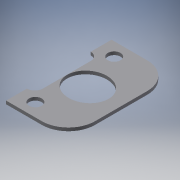
# Autodesk Inventor part: mocowanie_podwozia_dol
Saved by Autodesk Inventor 2017 (Build 210142000, 142)
## iProperties
Created: 2017-05-12
Part Number: mocowanie_podwozia_dol
Material: Ogólny
Document SubType Name: Modeling
Designer: Kuba01
Density: 1 g/cm^3
Appearance: Domyślna
Author: Kuba01
Autodesk Inventor part; units mm, degrees
ref_plane "YZ Plane" through (0, 0, 0) normal (1, 0, 0) x (0, 1, 0)
ref_plane "XZ Plane" through (0, 0, 0) normal (0, 1, 0) x (-1, 0, 0)
ref_plane "XY Plane" through (0, 0, 0) normal (0, 0, 1) x (1, 0, 0)
sketch "Szkic1" plane through (0, 0, 0) normal (0, 0, 1) x (1, 0, 0)
  arc A0 (-6.332, 7.5) -> (-8.832, 10) centre (-8.832, 7.5) ccw projected
  line L0 (-6.332, -7.5) -> (-6.332, 7.5) projected
  arc A1 (-8.832, -10) -> (-6.332, -7.5) centre (-8.832, -7.5) ccw projected
  line L1 (-8.832, -16.5118) -> (-8.832, -10) projected
  line L2 (2.345, -16.5118) -> (-8.832, -16.5118) projected
  arc A2 (2.345, -16.5118) -> (10.6894, -8.1674) centre (2.345, -8.1674) ccw projected
  line L3 (10.6894, 8.1674) -> (10.6894, -8.1674) projected
  arc A3 (10.6894, 8.1674) -> (2.345, 16.5118) centre (2.345, 8.1674) ccw projected
  line L4 (-8.832, 16.5118) -> (2.345, 16.5118) projected
  line L5 (-8.832, 10) -> (-8.832, 16.5118) projected
  circle A4 centre (-3.8436, 12.3396) radius 2 projected
  circle A5 centre (-3.8436, -12.3396) radius 2 projected
  ellipse E0 centre (0.246, 0) end of major axis (6.7679, 0) minor radius 6 projected
  point P0 (0, 0)
  constraints: 1 other
extrude "Wyciągnięcie proste1" add sketch "Szkic1" along normal blind 1
